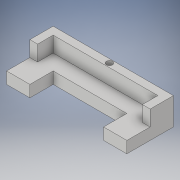
# Autodesk Inventor part: BatteryHolder
Saved by Autodesk Inventor 2019.4 (Build 234330000, 330)
## iProperties
Created: 2019-06-15
Part Number: BatteryHolder
Material: Generic
Document SubType Name: Modeling
Designer: steele
Density: 1 g/cm^3
Appearance: Default
Author: steele
Autodesk Inventor part; units mm, degrees
ref_plane "YZ Plane" through (0, 0, 0) normal (1, 0, 0) x (0, 1, 0)
ref_plane "XZ Plane" through (0, 0, 0) normal (0, 1, 0) x (-1, 0, 0)
ref_plane "XY Plane" through (0, 0, 0) normal (0, 0, 1) x (1, 0, 0)
sketch "Sketch1" plane through (0, 0, 0) normal (0, 1, 0) x (-1, 0, 0)
  line L0 (98.425, 38.1) -> (-98.425, 38.1)
  line L1 (-98.425, 38.1) -> (-98.425, -38.1)
  line L2 (-98.425, -38.1) -> (98.425, -38.1)
  line L3 (98.425, -38.1) -> (98.425, 38.1)
  line L4 (98.425, 38.1) -> (-98.425, -38.1) construction
  line L5 (-98.425, 38.1) -> (98.425, -38.1) construction
  point P0 (0, 0)
  dimension "length" = 196.85
  dimension "width" = 76.2
  constraints: 12 end point, 2 midpoint, 2 parallel, 1 horizontal, 1 perpendicular
  measures "length" distance of L0.start L0.end
  measures "width" distance of L1.end L0.end
extrude "Extrusion1" add sketch "Sketch1" along normal blind 19.05
sketch "Sketch3" plane through (0, 19.05, 0) normal (0, 1, 0) x (1, 0, 0)
  line L0 (98.425, 38.1) -> (-98.425, 38.1) projected
  line L1 (-98.425, 38.1) -> (98.425, 38.1)
  line L2 (98.425, 38.1) -> (98.425, 0)
  line L3 (98.425, -38.1) -> (98.425, 38.1) projected
  line L4 (98.425, 0) -> (85.725, 0)
  line L5 (85.725, 0) -> (85.725, 25.4)
  line L6 (85.725, 25.4) -> (-85.725, 25.4)
  line L7 (-85.725, 25.4) -> (-85.725, 0)
  line L8 (-85.725, 0) -> (-98.425, 0)
  line L9 (-98.425, 38.1) -> (-98.425, -38.1) projected
  line L10 (-98.425, 0) -> (-98.425, 38.1)
  point P0 (0, 0)
  dimension "d9" = 38.1
  dimension "batterSupportSideEdge" = 12.7
  dimension "batterySupportCutOut" = 25.4
  dimension "d28" = 12.7
  constraints: 16 end point, 4 perpendicular, 2 point on line, 1 collinear, 1 horizontal, 1 midpoint, 1 parallel
  measures "d9" distance of L0.start L2.end
  measures "batterSupportSideEdge" distance of L2.end L4.end
  measures "batterySupportCutOut" distance of L4.end L5.end
  measures "d28" distance between parallel lines of L9 L7
extrude "Extrusion2" add sketch "Sketch3" along normal blind 25.4
sketch "Sketch4" plane through (0, 44.45, 0) normal (0, 1, 0) x (1, 0, 0)
  line L0 (98.425, 38.1) -> (-98.425, 38.1) construction
  line L1 (0, 38.1) -> (0, 25.4) construction
  line L2 (-85.725, 25.4) -> (85.725, 25.4) projected
  point P0 (0, 0)
  point P1 (0, 31.75)
  dimension "d14" = 6.35
  constraints: 2 end point, 2 midpoint, 1 vertical
  measures "d14" distance from line of L2 point (0, 31.75)
hole "Hole1" at (0, 44.45, -31.75) direction (0, -1, 0) diameter 10.0838 end through all clearance for "Hex Head Bolt" size "3/8" standard "Ansi Unified Screw Threads"
sketch "Sketch5" plane through (0, 19.05, 0) normal (0, 1, 0) x (1, 0, 0)
  line L0 (-60.325, -38.1) -> (60.325, -38.1)
  line L1 (60.325, -38.1) -> (60.325, 0)
  line L2 (60.325, 0) -> (-60.325, 0)
  line L3 (-60.325, 0) -> (-60.325, -38.1)
  line L4 (-98.425, 0) -> (-98.425, -38.1) projected
  line L5 (98.425, -38.1) -> (98.425, 0) projected
  line L6 (85.725, 25.4) -> (-85.725, 25.4) projected
  point P0 (0, 0)
  dimension "d22" = 38.1
  dimension "d23" = 38.1
  dimension "d24" = 25.4
  constraints: 8 end point, 2 parallel, 1 horizontal, 1 perpendicular
  measures "d22" distance between parallel lines of L3 L4
  measures "d23" distance between parallel lines of L1 L5
  measures "d24" distance between parallel lines of L2 L6
extrude "Extrusion3" cut sketch "Sketch5" against normal through all
body "Solid1"
